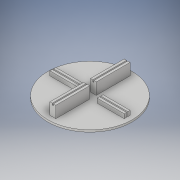
# Autodesk Inventor part: Soldering Jig
Saved by Autodesk Inventor 2018.3 (Build 223284000, 284)
## iProperties
Created: 2019-11-06
Part Number: Soldering Jig
Material: Generic
Document SubType Name: Modeling
Designer: Electro707
Density: 1 g/cm^3
Appearance: Default
Author: Electro707
Autodesk Inventor part; units mm, degrees
ref_plane "YZ Plane" through (0, 0, 0) normal (1, 0, 0) x (0, 1, 0)
ref_plane "XZ Plane" through (0, 0, 0) normal (0, 1, 0) x (-1, 0, 0)
ref_plane "XY Plane" through (0, 0, 0) normal (0, 0, 1) x (1, 0, 0)
sketch "Sketch1" plane through (0, 0, 0) normal (0, 1, 0) x (-1, 0, 0)
  line L0 (4.385, 55) -> (0.885, 55)
  line L1 (0.885, 55) -> (0.885, 5)
  line L2 (0.885, 5) -> (4.385, 5)
  line L3 (4.385, 5) -> (4.385, 55)
  line L4 (-0.865, 5) -> (-4.365, 5)
  line L5 (-4.365, 5) -> (-4.365, 55)
  line L6 (-4.365, 55) -> (-0.865, 55)
  line L7 (-0.865, 55) -> (-0.865, 5)
  line L8 (0.885, 5) -> (-0.865, 5)
  line L9 (-0.865, 55) -> (0.885, 55)
  line L10 (4.365, -5) -> (0.865, -5)
  line L11 (0.865, -5) -> (0.865, -55)
  line L12 (0.865, -55) -> (4.365, -55)
  line L13 (4.365, -55) -> (4.365, -5)
  line L14 (-0.885, -55) -> (-4.385, -55)
  line L15 (-4.385, -55) -> (-4.385, -5)
  line L16 (-4.385, -5) -> (-0.885, -5)
  line L17 (-0.885, -5) -> (-0.885, -55)
  line L18 (-0.885, -5) -> (0.865, -5)
  line L19 (0.865, -55) -> (-0.885, -55)
  line L20 (55, -4.375) -> (15, -4.375)
  line L21 (15, -4.375) -> (15, -0.875)
  line L22 (15, -0.875) -> (55, -0.875)
  line L23 (55, -0.875) -> (55, -4.375)
  line L24 (15, 0.875) -> (55, 0.875)
  line L25 (55, 0.875) -> (55, 4.375)
  line L26 (55, 4.375) -> (15, 4.375)
  line L27 (15, 4.375) -> (15, 0.875)
  line L28 (-15, -4.375) -> (-55, -4.375)
  line L29 (-55, -4.375) -> (-55, -0.875)
  line L30 (-55, -0.875) -> (-15, -0.875)
  line L31 (-15, -0.875) -> (-15, -4.375)
  line L32 (-55, 0.875) -> (-15, 0.875)
  line L33 (-15, 0.875) -> (-15, 4.375)
  line L34 (-15, 4.375) -> (-55, 4.375)
  line L35 (-55, 4.375) -> (-55, 0.875)
  line L36 (-15, 0.875) -> (-15, -0.875) construction
  line L37 (-55, -0.875) -> (-55, 0.875) construction
  line L38 (15, 0.875) -> (15, -0.875) construction
  line L39 (55, -0.875) -> (55, 0.875) construction
  line L40 (15, -4.375) -> (-15, -4.375) construction
  line L41 (-15, 4.375) -> (15, 4.375) construction
  line L42 (15, -4.375) -> (0, 0) construction
  line L43 (0, 0) -> (-15, -4.375) construction
  line L44 (-15, 4.375) -> (0, 0) construction
  line L45 (-4.385, -5) -> (0, 0) construction
  line L46 (0, 0) -> (4.385, 5) construction
  line L47 (0, 0) -> (4.365, -5) construction
  line L48 (0, 0) -> (-4.365, 5) construction
  point P0 (-0.01, -5)
  point P1 (0.01, 5)
  dimension "d0" = 1.75
  dimension "d2" = 110
  dimension "d3" = 3.5
  dimension "d5" = 40
  dimension "d15" = 30
  dimension "d16" = 10
  dimension "d21" = 0.01
  constraints: 98 end point, 17 equal length, 16 parallel, 10 horizontal, 8 perpendicular, 5 vertical, 4 point on line, 2 midpoint
  measures "d0" distance of L1.end L4.start
  measures "d2" distance between parallel lines of L0 L12
  measures "d3" distance of L0.start L0.end
  measures "d5" distance of L20.start L20.end
  measures "d15" distance of L20.end L28.start
  measures "d16" distance of L2.end L10.start
  measures "d21" horizontal distance of point (0.01, 5) L42.end
extrude "Extrusion1" add sketch "Sketch1" along normal blind 6.35 contours L20 L21 L22 L23 | L27 L26 L25 L24 | L28 L29 L30 L31 | L35 L34 L33 L32
extrude "Extrusion3" add sketch "Sketch1" along normal blind 17.25 contours L3 L2 L1 L0 | L7 L4 L5 L6 | L13 L12 L11 L10 | L17 L14 L15 L16
sketch "Sketch2" plane through (0, 0, 0) normal (0, -1, 0) x (1, 0, 0)
  circle A0 centre (0, 0) radius 62.23
  dimension "d8" = 124.46
  constraints: 1 centre point, 1 coincident
  measures "d8" diameter of A0
extrude "Extrusion2" add sketch "Sketch2" along normal blind 3
extrude "Extrusion4" add sketch "Sketch1" along normal blind 14.8 contours L3 L2 L1 L0 | L1 L8 L7 L9 | L7 L4 L5 L6 | L13 L12 L11 L10 | L11 L19 L17 L18 | L17 L14 L15 L16
body "Solid1"
